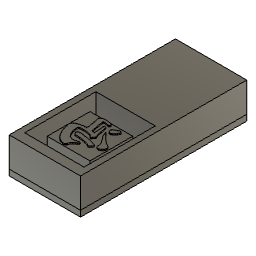
seal (Autodesk Fusion 360 design; units mm, degrees)
Autodesk Fusion 360 part; units mm, degrees
sketch "Sketch1" plane through (0, 0, 0) normal (0, 0, 1) x (1, 0, 0)
  line L0 (22.86, -22.86) -> (-22.86, -22.86)
  line L1 (-22.86, -22.86) -> (-22.86, 22.86)
  line L2 (-22.86, 22.86) -> (22.86, 22.86)
  line L3 (22.86, 22.86) -> (22.86, -22.86)
  line L4 (22.86, -22.86) -> (-22.86, 22.86) construction
  line L5 (-22.86, -22.86) -> (22.86, 22.86) construction
  line L6 (-38.1, -48.26) -> (38.1, -48.26)
  line L7 (38.1, -48.26) -> (38.1, 129.54)
  line L8 (38.1, 129.54) -> (-38.1, 129.54)
  line L9 (-38.1, 129.54) -> (-38.1, -48.26)
  line L10 (31.75, 38.1) -> (-31.75, 38.1)
  line L11 (-31.75, 38.1) -> (-31.75, -38.1)
  line L12 (-31.75, -38.1) -> (31.75, -38.1)
  line L13 (31.75, -38.1) -> (31.75, 38.1)
  line L14 (31.75, 38.1) -> (-31.75, -38.1) construction
  line L15 (-31.75, 38.1) -> (31.75, -38.1) construction
  line L16 (0, 129.54) -> (0, -48.26) construction
  dimension "d1" = 45.72
  dimension "d2" = 45.72
  dimension "d13" = 76.2
  dimension "d14" = 177.8
  dimension "d15" = 25.4
  dimension "d16" = 63.5
  dimension "d17" = 76.2
  constraint horizontal L0
  constraint perpendicular L0 L1
  constraint parallel L0 L2
  constraint parallel L1 L3
  constraint coincident L4 origin
  constraint coincident L5 origin
  constraint horizontal L6
  constraint vertical L7
  constraint horizontal L8
  constraint vertical L9
  constraint horizontal L10
  constraint perpendicular L10 L11
  constraint parallel L10 L12
  constraint parallel L11 L13
  constraint coincident L14 origin
  constraint coincident L15 origin
  constraint midpoint L8 L16.start
  constraint midpoint L6 L16.end
  constraint coincident origin L16
  measures "d1" distance of L1.end L2.end
  measures "d2" distance of L0.end L1.end
  measures "d13" distance of L6.start L6.end
  measures "d14" distance of L6.start L8.end
  measures "d15" distance of L0 L6
  measures "d16" distance of L11.end L12.end
  measures "d17" distance of L10.end L11.end
extrude "Extrude1" add sketch "Sketch1" along normal blind 25.4 contours L0 L1 L2 L3 makes body 1
sketch "Sketch2" plane through (0, 0, 25.4) normal (0, 0, 1) x (-1, 0, 0)
  line L0 (-22.86, -22.86) -> (22.86, -22.86)
  line L1 (22.86, -22.86) -> (22.86, 22.86)
  line L2 (22.86, 22.86) -> (-22.86, 22.86)
  line L3 (-22.86, 22.86) -> (-22.86, -22.86)
  spline S0 degree 2 poles (5.4753, 2.5018) (6.6856, 2.2885) (8.0549, 2.5487) knots 0 0 0 1 1 1
  spline S1 degree 2 poles (8.0549, 2.5487) (9.4768, 2.8088) (10.1096, 3.2812) knots 0 0 0 1 1 1
  spline S2 degree 2 poles (10.1096, 3.2812) (10.5315, 3.6487) (10.5846, 3.8592) knots 0 0 0 1 1 1
  spline S3 degree 2 poles (10.5846, 3.8592) (10.6904, 4.0695) (10.5867, 4.8068) knots 0 0 0 1 1 1
  spline S4 degree 2 poles (10.5867, 4.8068) (10.483, 5.4913) (10.273, 5.755) knots 0 0 0 1 1 1
  spline S5 degree 2 poles (10.273, 5.755) (10.1156, 6.0186) (9.5374, 6.3884) knots 0 0 0 1 1 1
  spline S6 degree 2 poles (9.5374, 6.3884) (8.7493, 7.0745) (8.1172, 6.9179) knots 0 0 0 1 1 1
  spline S7 degree 2 poles (8.1172, 6.9179) (7.4853, 6.814) (3.8536, 7.1379) knots 0 0 0 1 1 1
  spline S8 degree 2 poles (3.8536, 7.1379) (0.2745, 7.4091) (-0.3566, 7.6737) knots 0 0 0 1 1 1
  spline S9 degree 2 poles (-0.3566, 7.6737) (-1.0402, 7.991) (-2.5138, 8.2049) knots 0 0 0 1 1 1
  spline S10 degree 2 poles (-2.5138, 8.2049) (-6.5128, 9.0034) (-7.1429, 9.7417) knots 0 0 0 1 1 1
  spline S11 degree 2 poles (-7.1429, 9.7417) (-7.9825, 10.9544) (-9.0896, 10.2198) knots 0 0 0 1 1 1
  spline S12 degree 2 poles (-9.0896, 10.2198) (-9.8277, 9.7477) (-10.6193, 8.8545) knots 0 0 0 1 1 1
  spline S13 degree 2 poles (-10.6193, 8.8545) (-11.411, 7.9087) (-11.5702, 7.33) knots 0 0 0 1 1 1
  spline S14 degree 2 poles (-11.5702, 7.33) (-11.6764, 6.9091) (-11.5716, 6.6983) knots 0 0 0 1 1 1
  spline S15 degree 2 poles (-11.5716, 6.6983) (-11.4142, 6.4874) (-10.8883, 6.223) knots 0 0 0 1 1 1
  spline S16 degree 2 poles (-10.8883, 6.223) (-10.0472, 5.6947) (-9.1001, 5.482) knots 0 0 0 1 1 1
  spline S17 degree 2 poles (-9.1001, 5.482) (-8.1005, 5.2166) (-6.5223, 4.7393) knots 0 0 0 1 1 1
  spline S18 degree 2 poles (-6.5223, 4.7393) (-4.944, 4.2621) (-1.7339, 3.7812) knots 0 0 0 1 1 1
  spline S19 degree 2 poles (-1.7339, 3.7812) (1.4762, 3.3003) (1.634, 3.2473) knots 0 0 0 1 1 1
  spline S20 degree 2 poles (1.634, 3.2473) (1.7917, 3.1417) (3.16, 2.9281) knots 0 0 0 1 1 1
  spline S21 degree 2 poles (3.16, 2.9281) (4.5282, 2.7145) (5.4753, 2.5018) knots 0 0 0 1 1 1
  spline S22 degree 2 poles (-8.0295, -10.2605) (-6.5064, -11.8958) (-6.3485, -11.8961) knots 0 0 0 1 1 1
  spline S23 degree 2 poles (-6.3485, -11.8961) (-6.1906, -11.8965) (-6.1901, -11.6859) knots 0 0 0 1 1 1
  spline S24 degree 2 poles (-6.1901, -11.6859) (-6.137, -11.4755) (-6.2415, -11.1067) knots 0 0 0 1 1 1
  spline S25 degree 2 poles (-6.2415, -11.1067) (-6.3461, -10.7906) (-6.5558, -10.4217) knots 0 0 0 1 1 1
  spline S26 degree 2 poles (-6.5558, -10.4217) (-6.9754, -9.7364) (-7.2368, -8.8935) knots 0 0 0 1 1 1
  spline S27 degree 2 poles (-7.2368, -8.8935) (-7.8647, -7.1549) (-10.2797, -4.2016) knots 0 0 0 1 1 1
  spline S28 degree 2 poles (-10.2797, -4.2016) (-12.1693, -1.7232) (-13.4275, 0.6485) knots 0 0 0 1 1 1
  spline S29 degree 2 poles (-13.4275, 0.6485) (-14.6332, 2.9674) (-14.5253, 4.1253) knots 0 0 0 1 1 1
  spline S30 degree 2 poles (-14.5253, 4.1253) (-14.4699, 5.3886) (-14.6795, 5.8102) knots 0 0 0 1 1 1
  spline S31 degree 2 poles (-14.6795, 5.8102) (-14.8365, 6.2317) (-15.6777, 6.7074) knots 0 0 0 1 1 1
  spline S32 degree 2 poles (-15.6777, 6.7074) (-16.4663, 7.1829) (-16.7294, 7.2361) knots 0 0 0 1 1 1
  spline S33 degree 2 poles (-16.7294, 7.2361) (-16.9926, 7.2367) (-17.414, 7.1323) knots 0 0 0 1 1 1
  spline S34 degree 2 poles (-17.414, 7.1323) (-18.099, 6.818) (-19.1533, 6.1886) knots 0 0 0 1 1 1
  spline S35 degree 2 poles (-19.1533, 6.1886) (-20.155, 5.5065) (-20.3664, 5.1385) knots 0 0 0 1 1 1
  spline S36 degree 2 poles (-20.3664, 5.1385) (-20.7884, 4.7709) (-21.1585, 4.0347) knots 0 0 0 1 1 1
  spline S37 degree 2 poles (-21.1585, 4.0347) (-21.476, 3.2984) (-21.5294, 2.93) knots 0 0 0 1 1 1
  spline S38 degree 2 poles (-21.5294, 2.93) (-21.5831, 2.4564) (-21.742, 2.0356) knots 0 0 0 1 1 1
  spline S39 degree 2 poles (-21.742, 2.0356) (-21.8483, 1.562) (-21.6377, 1.5616) knots 0 0 0 1 1 1
  spline S40 degree 2 poles (-21.6377, 1.5616) (-21.4272, 1.5611) (-21.4277, 1.2979) knots 0 0 0 1 1 1
  spline S41 degree 2 poles (-21.4277, 1.2979) (-21.4283, 1.0347) (-21.0604, 0.7707) knots 0 0 0 1 1 1
  spline S42 degree 2 poles (-21.0604, 0.7707) (-20.6399, 0.5065) (-20.6404, 0.2433) knots 0 0 0 1 1 1
  spline S43 degree 2 poles (-20.6404, 0.2433) (-20.6411, -0.0726) (-19.8523, -0.4428) knots 0 0 0 1 1 1
  spline S44 degree 2 poles (-19.8523, -0.4428) (-14.8035, -2.665) (-8.0295, -10.2605) knots 0 0 0 1 1 1
  spline S45 degree 2 poles (-14.2082, -19.0908) (-13.5249, -19.5661) (-12.9458, -19.5673) knots 0 0 0 1 1 1
  spline S46 degree 2 poles (-12.9458, -19.5673) (-12.3667, -19.5686) (-10.8384, -18.7824) knots 0 0 0 1 1 1
  spline S47 degree 2 poles (-10.8384, -18.7824) (-9.2575, -18.0489) (-8.0447, -17.1566) knots 0 0 0 1 1 1
  spline S48 degree 2 poles (-8.0447, -17.1566) (-6.99, -16.3167) (-6.6732, -15.8962) knots 0 0 0 1 1 1
  spline S49 degree 2 poles (-6.6732, -15.8962) (-6.3564, -15.4758) (-6.5661, -15.0542) knots 0 0 0 1 1 1
  spline S50 degree 2 poles (-6.5661, -15.0542) (-6.7758, -14.6852) (-6.7747, -14.1588) knots 0 0 0 1 1 1
  spline S51 degree 2 poles (-6.7747, -14.1588) (-6.772, -12.948) (-8.6662, -12.5227) knots 0 0 0 1 1 1
  spline S52 degree 2 poles (-8.6662, -12.5227) (-9.4556, -12.4157) (-9.7188, -12.4151) knots 0 0 0 1 1 1
  spline S53 degree 2 poles (-9.7188, -12.4151) (-9.9821, -12.4672) (-10.5095, -12.8871) knots 0 0 0 1 1 1
  spline S54 degree 2 poles (-10.5095, -12.8871) (-11.3003, -13.4118) (-12.1445, -14.3049) knots 0 0 0 1 1 1
  spline S55 degree 2 poles (-12.1445, -14.3049) (-12.9363, -15.2507) (-13.3055, -15.5657) knots 0 0 0 1 1 1
  spline S56 degree 2 poles (-13.3055, -15.5657) (-13.6221, -15.9335) (-13.6226, -16.1441) knots 0 0 0 1 1 1
  spline S57 degree 2 poles (-13.6226, -16.1441) (-13.6232, -16.4073) (-14.2567, -17.2482) knots 0 0 0 1 1 1
  spline S58 degree 2 poles (-14.2567, -17.2482) (-14.8373, -17.9312) (-14.8381, -18.2997) knots 0 0 0 1 1 1
  spline S59 degree 2 poles (-14.8381, -18.2997) (-14.7864, -18.721) (-14.2082, -19.0908) knots 0 0 0 1 1 1
  spline S60 degree 2 poles (2.5782, -22.0759) (7.9467, -22.5616) (9.4237, -21.1961) knots 0 0 0 1 1 1
  spline S61 degree 2 poles (9.4237, -21.1961) (9.8983, -20.8287) (10.4255, -20.4613) knots 0 0 0 1 1 1
  spline S62 degree 2 poles (10.4255, -20.4613) (11.0054, -20.0941) (10.9543, -19.4097) knots 0 0 0 1 1 1
  spline S63 degree 2 poles (10.9543, -19.4097) (10.903, -18.7778) (10.0668, -16.0386) knots 0 0 0 1 1 1
  spline S64 degree 2 poles (10.0668, -16.0386) (9.8057, -15.0904) (9.8071, -14.4587) knots 0 0 0 1 1 1
  spline S65 degree 2 poles (9.8071, -14.4587) (9.8085, -13.827) (9.4943, -13.0893) knots 0 0 0 1 1 1
  spline S66 degree 2 poles (9.4943, -13.0893) (9.1801, -12.3516) (9.1825, -11.2461) knots 0 0 0 1 1 1
  spline S67 degree 2 poles (9.1825, -11.2461) (9.1848, -10.1933) (8.8711, -9.245) knots 0 0 0 1 1 1
  spline S68 degree 2 poles (8.8711, -9.245) (8.5573, -8.2968) (8.5083, -6.6647) knots 0 0 0 1 1 1
  line L4 (8.5083, -6.6647) -> (8.4593, -5.0327)
  line L5 (8.4593, -5.0327) -> (10.5652, -4.9321)
  spline S69 degree 2 poles (10.5652, -4.9321) (14.8827, -4.5731) (17.3595, -3.3678) knots 0 0 0 1 1 1
  spline S70 degree 2 poles (17.3595, -3.3678) (19.0986, -2.5294) (19.6258, -2.1621) knots 0 0 0 1 1 1
  spline S71 degree 2 poles (19.6258, -2.1621) (20.1531, -1.7947) (20.7865, -1.0065) knots 0 0 0 1 1 1
  spline S72 degree 2 poles (20.7865, -1.0065) (22.2122, 0.9381) (21.6344, 1.5185) knots 0 0 0 1 1 1
  spline S73 degree 2 poles (21.6344, 1.5185) (21.4244, 1.7822) (21.2689, 2.888) knots 0 0 0 1 1 1
  spline S74 degree 2 poles (21.2689, 2.888) (21.1135, 3.9938) (20.8505, 4.0997) knots 0 0 0 1 1 1
  spline S75 degree 2 poles (20.8505, 4.0997) (20.5875, 4.2056) (20.5904, 5.5216) knots 0 0 0 1 1 1
  spline S76 degree 2 poles (20.5904, 5.5216) (20.5933, 6.8377) (20.2778, 6.9963) knots 0 0 0 1 1 1
  spline S77 degree 2 poles (20.2778, 6.9963) (19.9622, 7.1023) (19.9638, 7.8393) knots 0 0 0 1 1 1
  spline S78 degree 2 poles (19.9638, 7.8393) (19.965, 8.3657) (19.5981, 9.1035) knots 0 0 0 1 1 1
  spline S79 degree 2 poles (19.5981, 9.1035) (19.2839, 9.8412) (17.9215, 12.6869) knots 0 0 0 1 1 1
  spline S80 degree 2 poles (17.9215, 12.6869) (16.663, 14.9007) (15.9809, 15.9551) knots 0 0 0 1 1 1
  spline S81 degree 2 poles (15.9809, 15.9551) (15.2988, 16.9568) (13.9857, 18.2757) knots 0 0 0 1 1 1
  spline S82 degree 2 poles (13.9857, 18.2757) (12.4622, 19.7005) (11.2003, 20.3876) knots 0 0 0 1 1 1
  spline S83 degree 2 poles (11.2003, 20.3876) (9.991, 21.0746) (7.7812, 21.606) knots 0 0 0 1 1 1
  spline S84 degree 2 poles (7.7812, 21.606) (6.4657, 21.8721) (6.0972, 21.8729) knots 0 0 0 1 1 1
  spline S85 degree 2 poles (6.0972, 21.8729) (5.7814, 21.8736) (5.5705, 21.7161) knots 0 0 0 1 1 1
  spline S86 degree 2 poles (5.5705, 21.7161) (5.3591, 21.3481) (5.2011, 21.3485) knots 0 0 0 1 1 1
  spline S87 degree 2 poles (5.2011, 21.3485) (5.0432, 21.3488) (4.6208, 20.7707) knots 0 0 0 1 1 1
  spline S88 degree 2 poles (4.6208, 20.7707) (4.2511, 20.2451) (4.1447, 19.7189) knots 0 0 0 1 1 1
  spline S89 degree 2 poles (4.1447, 19.7189) (3.9319, 18.7191) (3.562, 18.0882) knots 0 0 0 1 1 1
  spline S90 degree 2 poles (3.562, 18.0882) (3.1921, 17.4573) (2.2426, 16.5645) knots 0 0 0 1 1 1
  spline S91 degree 2 poles (2.2426, 16.5645) (1.0818, 15.3563) (0.5545, 14.989) knots 0 0 0 1 1 1
  spline S92 degree 2 poles (0.5545, 14.989) (0.0798, 14.5689) (-0.7636, 14.0443) knots 0 0 0 1 1 1
  spline S93 degree 2 poles (-0.7636, 14.0443) (-2.2922, 13.1528) (-1.9254, 12.415) knots 0 0 0 1 1 1
  spline S94 degree 2 poles (-1.9254, 12.415) (-1.6109, 11.7826) (0.4436, 12.4624) knots 0 0 0 1 1 1
  spline S95 degree 2 poles (0.4436, 12.4624) (3.6047, 13.6135) (5.6573, 13.3984) knots 0 0 0 1 1 1
  spline S96 degree 2 poles (5.6573, 13.3984) (7.7098, 13.1307) (9.4435, 11.5475) knots 0 0 0 1 1 1
  spline S97 degree 2 poles (9.4435, 11.5475) (11.0196, 10.1227) (12.2238, 7.1194) knots 0 0 0 1 1 1
  spline S98 degree 2 poles (12.2238, 7.1194) (12.5375, 6.1712) (12.8519, 5.4861) knots 0 0 0 1 1 1
  spline S99 degree 2 poles (12.8519, 5.4861) (13.1662, 4.8011) (13.1646, 4.0641) knots 0 0 0 1 1 1
  spline S100 degree 2 poles (13.1646, 4.0641) (13.1629, 3.3271) (13.4762, 2.1682) knots 0 0 0 1 1 1
  spline S101 degree 2 poles (13.4762, 2.1682) (14.0503, -0.0967) (13.2593, -0.7266) knots 0 0 0 1 1 1
  spline S102 degree 2 poles (13.2593, -0.7266) (12.7319, -1.1466) (12.0472, -1.303) knots 0 0 0 1 1 1
  spline S103 degree 2 poles (12.0472, -1.303) (11.3625, -1.4594) (8.7829, -1.5064) knots 0 0 0 1 1 1
  spline S104 degree 2 poles (8.7829, -1.5064) (4.2028, -1.6015) (1.6777, -0.8063) knots 0 0 0 1 1 1
  spline S105 degree 2 poles (1.6777, -0.8063) (-0.7947, -0.0112) (-2.2642, 2.0451) knots 0 0 0 1 1 1
  spline S106 degree 2 poles (-2.2642, 2.0451) (-2.4215, 2.3087) (-2.5795, 2.309) knots 0 0 0 1 1 1
  spline S107 degree 2 poles (-2.5795, 2.309) (-2.6847, 2.3093) (-3.0013, 1.9941) knots 0 0 0 1 1 1
  spline S108 degree 2 poles (-3.0013, 1.9941) (-3.4235, 1.5213) (-3.4239, 1.3107) knots 0 0 0 1 1 1
  spline S109 degree 2 poles (-3.4239, 1.3107) (-3.425, 0.8369) (-4.7968, -0.5814) knots 0 0 0 1 1 1
  spline S110 degree 2 poles (-4.7968, -0.5814) (-5.1661, -0.9491) (-5.1675, -1.5808) knots 0 0 0 1 1 1
  spline S111 degree 2 poles (-5.1675, -1.5808) (-5.1689, -2.2125) (-4.8013, -2.5818) knots 0 0 0 1 1 1
  spline S112 degree 2 poles (-4.8013, -2.5818) (-4.4863, -3.0036) (-4.4868, -3.2142) knots 0 0 0 1 1 1
  spline S113 degree 2 poles (-4.4868, -3.2142) (-4.4873, -3.4248) (-4.2767, -3.4252) knots 0 0 0 1 1 1
  spline S114 degree 2 poles (-4.2767, -3.4252) (-3.8556, -3.4262) (-2.9724, -8.745) knots 0 0 0 1 1 1
  spline S115 degree 2 poles (-2.9724, -8.745) (-2.2968, -12.6947) (-1.9311, -13.959) knots 0 0 0 1 1 1
  spline S116 degree 2 poles (-1.9311, -13.959) (-1.5655, -15.2758) (-1.1977, -15.5925) knots 0 0 0 1 1 1
  spline S117 degree 2 poles (-1.1977, -15.5925) (-0.7246, -15.9094) (-0.0928, -15.8582) knots 0 0 0 1 1 1
  spline S118 degree 2 poles (-0.0928, -15.8582) (0.3286, -15.7538) (0.4341, -15.6488) knots 0 0 0 1 1 1
  spline S119 degree 2 poles (0.4341, -15.6488) (0.5922, -15.5438) (0.6463, -14.9122) knots 0 0 0 1 1 1
  spline S120 degree 2 poles (0.6463, -14.9122) (0.7533, -14.1228) (0.4392, -13.3325) knots 0 0 0 1 1 1
  spline S121 degree 2 poles (0.4392, -13.3325) (0.0216, -11.7523) (-0.2293, -6.1716) knots 0 0 0 1 1 1
  spline S122 degree 2 poles (-0.2293, -6.1716) (-0.3836, -4.5394) (-0.0676, -4.4874) knots 0 0 0 1 1 1
  spline S123 degree 2 poles (-0.0676, -4.4874) (-0.015, -4.4875) (0.1428, -4.5405) knots 0 0 0 1 1 1
  spline S124 degree 2 poles (0.1428, -4.5405) (0.6162, -4.6995) (1.6687, -4.8597) knots 0 0 0 1 1 1
  line L6 (1.6687, -4.8597) -> (2.6161, -4.9671)
  line L7 (2.6161, -4.9671) -> (2.9818, -6.2314)
  spline S125 degree 2 poles (2.9818, -6.2314) (3.4001, -7.4957) (3.4508, -8.3907) knots 0 0 0 1 1 1
  line L8 (3.4508, -8.3907) -> (4.0229, -11.5506)
  spline S126 degree 2 poles (4.0229, -11.5506) (4.8544, -16.3955) (4.9556, -18.2382) knots 0 0 0 1 1 1
  line L9 (4.9556, -18.2382) -> (5.0054, -19.5544)
  line L10 (5.0054, -19.5544) -> (3.3209, -19.4981)
  spline S127 degree 2 poles (3.3209, -19.4981) (1.584, -19.3889) (0.3741, -18.9651) knots 0 0 0 1 1 1
  spline S128 degree 2 poles (0.3741, -18.9651) (-0.6253, -18.5944) (-1.0992, -18.646) knots 0 0 0 1 1 1
  spline S129 degree 2 poles (-1.0992, -18.646) (-1.5205, -18.7503) (-1.9957, -19.381) knots 0 0 0 1 1 1
  spline S130 degree 2 poles (-1.9957, -19.381) (-2.3653, -19.854) (-2.3137, -20.3279) knots 0 0 0 1 1 1
  spline S131 degree 2 poles (-2.3137, -20.3279) (-2.2621, -20.8018) (-1.7883, -20.8028) knots 0 0 0 1 1 1
  spline S132 degree 2 poles (-1.7883, -20.8028) (-1.4198, -20.8036) (-1.4204, -21.0668) knots 0 0 0 1 1 1
  spline S133 degree 2 poles (-1.4204, -21.0668) (-1.4209, -21.2774) (-0.2108, -21.5959) knots 0 0 0 1 1 1
  spline S134 degree 2 poles (-0.2108, -21.5959) (1.0518, -21.9672) (2.5782, -22.0759) knots 0 0 0 1 1 1
extrude "Extrude5" add sketch "Sketch2" along normal blind 1.27 separate body contours S0 S1 S2 S3 S4 S5 S6 S7 S8 S9 S10 S11 S12 S13 S14 S15 S16 S17 S18 S19 S20 S21 | S22 S23 S24 S25 S26 S27 S28 S29 S30 S31 S32 S33 S34 S35 S36 S37 S38 S39 S40 S41 S42 S43 S44 | S45 S46 S47 S48 S49 S50 S51 S52 S53 S54 S55 S56 S57 S58 S59 | S60 S61 S62 S63 S64 S65 S66 S67 S68 L4 L5 S69 S70 S71 S72 S73 S74 S75 S76 S77 S78 S79 S80 S81 S82 S83 S84 S85 S86 S87 S88 S89 S90 S91 S92 S93 S94 S95 S96 S97 S98 S99 S100 S101 S102 S103 S104 S105 S106 S107 S108 S109 S110 S111 S112 S113 S114 S115 S116 S117 S118 S119 S120 S121 S122 S123 S124 L6 L7 S125 L8 S126 L9 L10 S127 S128 S129 S130 S131 S132 S133 S134 makes body 2 at (-0.0144, -4.8565, 25.4) makes body 3 at (18.5061, -2.9125, 25.4) makes body 4 at (-6.2619, 14.7492, 25.4) makes body 5 at (8.438, 14.8254, 25.4)
extrude "Extrude6" add sketch "Sketch1" along normal blind 31.75 separate body contours L6 L7 L8 L9 makes body 6
extrude "Extrude7" add sketch "Sketch1" against normal blind 6.35 separate body contours L0 L1 L2 L3 | L6 L7 L8 L9 | L10 L11 L12 L13 makes body 7
move_body "Move5" bodies 2 to x (1, 0, 0) y (0, 1, 0) z (0, 0, 1) at (0.508, -0.635, 0)
move_body "Move6" bodies 3 to x (1, 0, 0) y (0, 1, 0) z (0, 0, 1) at (0, -1.27, 0)
